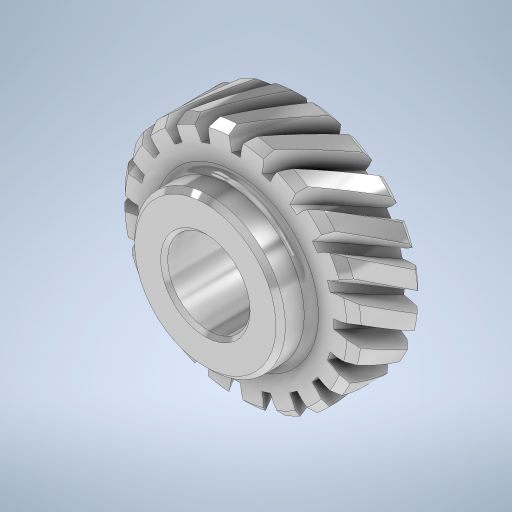
# Autodesk Inventor part: Engrenagem Helicoidal
Saved by Autodesk Inventor 2023 (Build 270158030, 158C)
## iProperties
Created: 2022-07-18
Part Number: Engrenagem Helicoidal
Material: Generic
Document SubType Name: Modeling
Designer: coqui
Density: 1 g/cm^3
Appearance: Chrome - Polished
Author: coqui
Autodesk Inventor part; units mm, degrees
ref_plane "YZ Plane" through (0, 0, 0) normal (1, 0, 0) x (0, 1, 0)
ref_plane "XZ Plane" through (0, 0, 0) normal (0, 1, 0) x (-1, 0, 0)
ref_plane "XY Plane" through (0, 0, 0) normal (0, 0, 1) x (1, 0, 0)
sketch "Sketch1" plane through (0, 0, 0) normal (0, 1, 0) x (-1, 0, 0)
  line L0 (0, 34.051) -> (0, -42.8) construction
  line L1 (-28.6196, 0) -> (27.8293, 0) construction
  line L2 (19, -15) -> (47.19, -15)
  line L3 (50.19, -12) -> (50.19, 12)
  line L4 (47.19, 15) -> (35, 15)
  line L5 (32, 18) -> (32, 26)
  line L6 (30, 28) -> (19, 28)
  line L7 (17.5, 26.5) -> (17.5, -13.5)
  arc A0 (32, 18) -> (35, 15) centre (35, 18) ccw
  line L8 (32, 26) -> (30, 28)
  line L9 (47.19, 15) -> (50.19, 12)
  line L10 (50.19, -12) -> (47.19, -15)
  line L11 (19, -15) -> (17.5, -13.5)
  line L12 (19, 28) -> (17.5, 26.5)
  point P0 (0, 0)
  point P1 (17.5, -15)
  point P2 (50.19, -15)
  point P3 (50.19, 15)
  point P4 (32, 15)
  point P5 (32, 28)
  point P6 (17.5, 28)
  point P7 (-0.3952, 0)
  dimension "d0" = 43
  dimension "d1" = 30
  dimension "d2" = 32.69
  dimension "d3" = 18.19
  dimension "d6" = 17.5
  dimension "d7" = 15
  dimension "d8" = 3
  dimension "d9" = 2
  dimension "d10" = 2
  dimension "d11" = 3
  dimension "d12" = 3
  dimension "d13" = 3
  dimension "d14" = 3
  dimension "d15" = 1.5
  dimension "d16" = 1.5
  dimension "d17" = 1.5
  dimension "d18" = 1.5
  constraints: 26 end point, 12 point on line, 5 perpendicular, 3 horizontal, 2 point on circle, 2 tangent, 2 vertical, 1 centre point, 1 midpoint
  measures "d0" distance of point (17.5, 28) point (17.5, -15)
  measures "d1" distance of point (50.19, -15) point (50.19, 15)
  measures "d2" distance of point (17.5, -15) point (50.19, -15)
  measures "d3" distance of point (50.19, 15) point (32, 15)
  measures "d6" distance from line of L0 point (17.5, -15)
  measures "d7" distance from line of L1 point (17.5, -15)
  measures "d8" radius of A0
  measures "d9" distance of L5.end point (32, 28)
  measures "d10" distance of L6.start point (32, 28)
  measures "d11" distance of L4.start point (50.19, 15)
  measures "d12" distance of L3.end point (50.19, 15)
  measures "d13" distance of L3.start point (50.19, -15)
  measures "d14" distance of L2.end point (50.19, -15)
  measures "d15" distance of L2.start point (17.5, -15)
  measures "d16" distance of L7.end point (17.5, -15)
  measures "d17" distance of L6.end point (17.5, 28)
  measures "d18" distance of L7.start point (17.5, 28)
revolve "Revolution1" add sketch "Sketch1" angle 360 about axis through (0, 0, 34.051) along (0, 0, -1)
sketch "Sketch2" plane through (0, 0, 15) normal (0, 0, 1) x (1, 0, 0)
  arc A0 (1.8974, 41.4566) -> (-1.8974, 41.4566) centre (0, 0) ccw
  arc A1 (5.1536, 51.4425) -> (-5.1536, 51.4425) centre (0, 0) ccw
  arc A2 (5.1536, 51.4425) -> (1.8974, 41.4566) centre (21.8729, 40.4668) ccw
  line L0 (0, 59.7913) -> (0, -67.5729) construction
  arc A3 (-1.8974, 41.4566) -> (-5.1536, 51.4425) centre (-21.8729, 40.4668) ccw
  point P0 (7.147, 54)
  point P1 (1.88, 41)
  point P2 (-7.147, 54)
  point P3 (-1.88, 41)
  dimension "d20" = 83
  dimension "d21" = 103.4
  dimension "d22" = 7.147
  dimension "d23" = 20
  dimension "d24" = 41
  dimension "d25" = 1.88
  dimension "d26" = 13
  constraints: 8 point on circle, 4 centre point, 3 symmetric about line, 2 coincident, 2 end point, 2 vertical, 1 other
  measures "d20" diameter of A0
  measures "d21" diameter of A1
  measures "d22" distance from line of point (7.147, 54) L0
  measures "d23" radius of A2
  measures "d24" vertical distance of point (0, 0) point (1.88, 41)
  measures "d25" distance from line of point (1.88, 41) L0
  measures "d26" vertical distance of point (1.88, 41) point (7.147, 54)
sketch "Sketch3" plane through (0, 0, 0) normal (0, 1, 0) x (-1, 0, 0)
  line L0 (0, 72.7214) -> (0, -58.8589) construction
  point P0 (0, 0)
  constraints: 2 end point, 1 vertical
coil "Coil1" sketch "Sketch2" operation cut axis through (0, 0, 72.7214) along (0, 0, -1) pitch 502.65 turns 0.059684 hand right
pattern_circular "Circular Pattern1" count 20 over 360 about axis through (0, 0, 6.5) along (0, 0, -1) of "Coil1"
equation "\"d10\" = d9"
equation "\"d12\" = d11"
equation "\"d13\" = d11"
equation "\"d14\" = d13"
equation "\"d16\" = d15"
equation "\"d17\" = d15"
equation "\"d18\" = d17"
body "Solid1"
